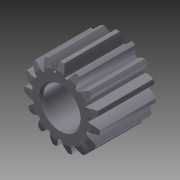
# Autodesk Inventor part: 15T Gear P60 Pinion Gear
Saved by Autodesk Inventor 2014 SP1 (Build 180222100, 222)
## iProperties
Created: 2013-05-05
Part Number: 15T Gear P60 Pinion Gear
Material: Steel
Document SubType Name: Modeling
Designer: Moses
Categories: <?xml version="1.0" encoding="UTF-16"?> <MemberInstance><Categories><FamilyTemplate><FamilyTemplateParameter ValueType="xs:double" Id="1" ObjectReferenceKey="da_z" ObjectType="kUserParameterObject"/><FamilyTemplateParameter ValueType="xs:double" Id="2" ObjectReferenceKey="da_b" ObjectType="kUserParameterObject"/><FamilyTemplateParameter ValueType="xs:double" Id="3" ObjectReferenceKey="da_beta" ObjectType="kUserParameterObject"/><FamilyTemplateParameter ValueType="xs:double" Id="4" ObjectReferenceKey="da_da" ObjectType="kUserParameterObject"/><FamilyTemplateParameter ValueType="xs:double" Id="5" ObjectReferenceKey="da_aw" ObjectType="kUserParameterObject"/><FamilyTemplateParameter ValueType="xs:string" Id="6" ObjectReferenceKey="EAIAABAAAAC/AAAAAAAAAIAAAAAAAAAA" ObjectType="83910656" SubObjectId="SurfaceGeometry"/></FamilyTemplate><ParamToTemplateMap><ParamToTemplate CategoryParameter="//CategoryParameter[@InternalName='046C89C9-8512-4d59-83FE-43B91F4F132A']" TemplateParameter="1"/><ParamToTemplate CategoryParameter="//CategoryParameter[@InternalName='2552DF32-E462-4b46-AEBF-C6C7768E72AC']" TemplateParameter="2"/><ParamToTemplate CategoryParameter="//CategoryParameter[@InternalName='C9EE641D-15FC-4fae-A226-E94C4372FDD7']" TemplateParameter="3"/><ParamToTemplate><ParamToTemplate CategoryParameter="//CategoryParameter[@InternalName='00B6519A-459B-49c7-AD84-2E56D39A5744']" ConstantValue="0.000000"/></ParamToTemplate><ParamToTemplate><ParamToTemplate CategoryParameter="//CategoryParameter[@InternalName='04B31F0E-C7A6-4894-AA32-9629BEFACF47']" ConstantValue="1.000000"/></ParamToTemplate><ParamToTemplate><ParamToTemplate CategoryParameter="//CategoryParameter[@InternalName='43CBEC2E-7847-49e7-A936-2F7889FCB2D9']" ConstantValue="0.250000"/></ParamToTemplate><ParamToTemplate><ParamToTemplate CategoryParameter="//CategoryParameter[@InternalName='B1EFC894-105D-4ebd-86BF-FA20ED196853']" ConstantValue="0.350000"/></ParamToTemplate><ParamToTemplate><ParamToTemplate CategoryParameter="//CategoryParameter[@InternalName='51175063-3D10-4879-93E8-6246FE8B403D']" ConstantValue="2060110000.000000"/></ParamToTemplate><ParamToTemplate><ParamToTemplate CategoryParameter="//CategoryParameter[@InternalName='A3A52E27-4454-46a9-B0BD-C932399B70AF']" ConstantValue="0.300000"/></ParamToTemplate><ParamToTemplate><ParamToTemplate CategoryParameter="//CategoryParameter[@InternalName='91B76062-C214-41d9-B1B9-14D2AB99603D']" ConstantValue="0.060000"/></ParamToTemplate><ParamToTemplate><ParamToTemplate CategoryParameter="//CategoryParameter[@InternalName='374E806E-8B8A-4dda-A9AA-1039D6500AD2']" ConstantValue="16.666667"/></ParamToTemplate><ParamToTemplate><ParamToTemplate CategoryParameter="//CategoryParameter[@InternalName='2D373A89-B862-43d6-8D0B-0CBF12AB9F6C']" ConstantValue="0.349066"/></ParamToTemplate><ParamToTemplate CategoryParameter="//CategoryParameter[@InternalName='37777632-D6A2-4fac-9D53-DB8ACD95C989']" TemplateParameter="4"/><ParamToTemplate CategoryParameter="//CategoryParameter[@InternalName='FD1017F1-B727-4f7e-9707-0F86F1FF9423']" TemplateParameter="5"/><ParamToTemplate><ParamToTemplate CategoryParameter="//CategoryParameter[@InternalName='9E1B4470-B2D3-4ff1-B813-535BB4CDF51A']" ConstantValue="3520790.000000"/></ParamToTemplate><ParamToTemplate><ParamToTemplate CategoryParameter="//CategoryParameter[@InternalName='F8452263-BFF6-458c-9FB1-07C4B99E95CD']" ConstantValue="11389170.000000"/></ParamToTemplate><ParamToTemplate><ParamToTemplate CategoryParameter="//CategoryParameter[@InternalName='3E3BB259-FD49-497f-8171-6EBC954A3479']" ConstantValue="2.000000"/></ParamToTemplate><ParamToTemplate CategoryParameter="//CategoryParameter[@InternalName='27C3BAF2-7550-4e4b-AE2C-0DB134B7D9B7']" TemplateParameter="6"/></ParamToTemplateMap><Category DisplayName="Gear" InternalName="DC85795E-93AB-48d5-8EEE-5A27447B64BD" Mnemonic="Gear"><CategoryParameter DisplayName="z" InternalName="046C89C9-8512-4d59-83FE-43B91F4F132A" Mnemonic="z"/><CategoryParameter DisplayName="b" InternalName="2552DF32-E462-4b46-AEBF-C6C7768E72AC" Mnemonic="b"/><CategoryParameter DisplayName="||b|" InternalName="C9EE641D-15FC-4fae-A226-E94C4372FDD7" Mnemonic="beta"/><CategoryParameter DisplayName="x" InternalName="00B6519A-459B-49c7-AD84-2E56D39A5744" Mnemonic="x"/><CategoryParameter DisplayName="a*" InternalName="04B31F0E-C7A6-4894-AA32-9629BEFACF47" Mnemonic="a"/><CategoryParameter DisplayName="c*" InternalName="43CBEC2E-7847-49e7-A936-2F7889FCB2D9" Mnemonic="c"/><CategoryParameter DisplayName="r|.f|*" InternalName="B1EFC894-105D-4ebd-86BF-FA20ED196853" Mnemonic="rf"/><CategoryParameter DisplayName="E" InternalName="51175063-3D10-4879-93E8-6246FE8B403D" Mnemonic="E"/><CategoryParameter DisplayName="||m|" InternalName="A3A52E27-4454-46a9-B0BD-C932399B70AF" Mnemonic="mi"/><Category DisplayName="SpurGear" InternalName="26C5A22E-A91E-4dfd-A3B3-23CCAFAE1764" Mnemonic="SpurGear"><CategoryParameter DisplayName="m" InternalName="91B76062-C214-41d9-B1B9-14D2AB99603D" Mnemonic="m"/><CategoryParameter DisplayName="P" InternalName="374E806E-8B8A-4dda-A9AA-1039D6500AD2" Mnemonic="PP"/><CategoryParameter DisplayName="||a|" InternalName="2D373A89-B862-43d6-8D0B-0CBF12AB9F6C" Mnemonic="alpha"/><CategoryParameter DisplayName="d|.a|" InternalName="37777632-D6A2-4fac-9D53-DB8ACD95C989" Mnemonic="da"/><CategoryParameter DisplayName="a|.w|" InternalName="FD1017F1-B727-4f7e-9707-0F86F1FF9423" Mnemonic="aw"/><CategoryParameter DisplayName="||s||.Flim|" InternalName="9E1B4470-B2D3-4ff1-B813-535BB4CDF51A" Mnemonic="sFlim"/><CategoryParameter DisplayName="||s||.Hlim|" InternalName="F8452263-BFF6-458c-9FB1-07C4B99E95CD" Mnemonic="sHlim"/><CategoryParameter DisplayName="type" InternalName="3E3BB259-FD49-497f-8171-6EBC954A3479" Mnemonic="type"/><CategoryParameter DisplayName="PitchDiameter" InternalName="27C3BAF2-7550-4e4b-AE2C-0DB134B7D9B7" Mnemonic="IDS_PITCHDIAM"/></Category></Category></Categories></MemberInstance>
Density: 7.85 g/cm^3
Mass: 2.25857 g
Surface Area: 4.2591 cm^2
Volume: 0.287716 cm^3
Appearance: Steel
CustomPartVersion: 1
Author: Moses
Autodesk Inventor part; units mm, degrees
sketch "Sketch1" plane through (0, 0, 0) normal (0, 0, 1) x (1, 0, 0)
  circle A0 centre (0, 0) radius 5.1
  dimension "d0" = 10.2
  constraints: 1 centre point
  measures "d0" diameter of A0
extrude "Extrusion1" add sketch "Sketch1" along normal mid plane 5
sketch "Sketch2" plane through (0, 0, -2.5) normal (0, 0, -1) x (-1, 0, 0)
  circle A0 centre (0, 0) radius 5.1 projected
  circle A1 centre (0, 0) radius 4.5
  dimension "d3" = 9
  constraints: 1 centre point, 1 coincident
  measures "d3" diameter of A1
surface extrude "Pitch Diameter" sketch "Sketch2" against normal through all shown no curves A1
ref_plane "Work Plane1" through (0, 0, 0) normal (1, 0, 0) x (0, 1, 0)
ref_plane "Work Plane2" through (0, 0, 0) normal (0.9781476, 0.2079117, 0) x (0, 0, 1)
ref_plane "Work Plane3" through (0, 0, 0) normal (0, 0, -1) x (-1, 0, 0)
spur gear teeth "Spur Gear" teeth 15 pitch diameter 9 tip diameter 10.2 root diameter 7.5 face width 5 start plane through (0, 0, -2.5) normal (0, 0, -1) x (-1, 0, 0)
sketch "Sketch3" plane through (0, 0, 2.5) normal (0, 0, 1) x (1, 0, 0)
  arc A0 (-1.8277, 4.7613) -> (-2.3154, 4.5441) centre (0, 0) ccw projected
  circle A1 centre (0, 0) radius 2.5
  dimension "d20" = 5
  constraints: 1 centre point, 1 coincident
  measures "d20" diameter of A1
extrude "Extrusion2" cut sketch "Sketch3" against normal through all
chamfer "Chamfer3" distance 1 angle 15 15 edges at (4.8504, 1.576, -2.5) (5.0721, -0.5331, -2.5) (3.79, 3.4126, -2.5) (4.4167, -2.55, -2.5) (2.0744, 4.6591, -2.5) (2.9977, -4.126, -2.5) (0, 5.1, -2.5) (1.0603, -4.9886, -2.5) (-2.0744, 4.6591, -2.5) (-1.0603, -4.9886, -2.5) (-3.79, 3.4126, -2.5) (-2.9977, -4.126, -2.5) (-4.8504, 1.576, -2.5) (-4.4167, -2.55, -2.5) (-5.0721, -0.5331, -2.5) measured on face at (-0.1004, 3.2965, -2.5)
sketch "Sketch4" plane through (0, 0, 2.5) normal (0, 0, 1) x (1, 0, 0)
  arc A0 (-2.36, 2.9143) -> (-3.6062, 3.6062) centre (-5.0149, -0.3993) ccw projected
  arc A1 (-3.6062, 3.6062) -> (-3.9634, 3.2095) centre (0, 0) ccw projected
  arc A2 (-3.9634, 3.2095) -> (-3.145, 2.0424) centre (-0.1271, 5.0291) ccw projected
  arc A3 (-3.145, 2.0424) -> (-3.3413, 1.7025) centre (0, 0) ccw projected
  arc A4 (-3.3413, 1.7025) -> (-4.7613, 1.8277) centre (-4.4189, -2.4045) ccw projected
  arc A5 (-4.7613, 1.8277) -> (-4.9262, 1.32) centre (0, 0) ccw projected
  arc A6 (-4.9262, 1.32) -> (-3.7038, 0.5866) centre (-2.1617, 4.5426) ccw projected
  arc A7 (-3.7038, 0.5866) -> (-3.7449, 0.1963) centre (0, 0) ccw projected
  arc A8 (-3.7449, 0.1963) -> (-5.093, -0.2669) centre (-3.0589, -3.9939) ccw projected
  arc A9 (-5.093, -0.2669) -> (-5.0372, -0.7978) centre (0, 0) ccw projected
  arc A10 (-5.0372, -0.7978) -> (-3.6222, -0.9706) centre (-3.8224, 3.2707) ccw projected
  arc A11 (-3.6222, -0.9706) -> (-3.5009, -1.3439) centre (0, 0) ccw projected
  arc A12 (-3.5009, -1.3439) -> (-4.5441, -2.3154) centre (-1.17, -4.8928) ccw projected
  arc A13 (-4.5441, -2.3154) -> (-4.2772, -2.7777) centre (0, 0) ccw projected
  arc A14 (-4.2772, -2.7777) -> (-2.9143, -2.36) centre (-4.8223, 1.4332) ccw projected
  arc A15 (-2.9143, -2.36) -> (-2.6517, -2.6517) centre (0, 0) ccw projected
  arc A16 (-2.6517, -2.6517) -> (-3.2095, -3.9634) centre (0.9213, -4.9457) ccw projected
  arc A17 (-3.2095, -3.9634) -> (-2.7777, -4.2772) centre (0, 0) ccw projected
  arc A18 (-2.7777, -4.2772) -> (-1.7025, -3.3413) centre (-4.9883, -0.6521) ccw projected
  arc A19 (-1.7025, -3.3413) -> (-1.3439, -3.5009) centre (0, 0) ccw projected
  arc A20 (-1.3439, -3.5009) -> (-1.32, -4.9262) centre (2.8532, -4.1434) ccw projected
  arc A21 (-1.32, -4.9262) -> (-0.7978, -5.0372) centre (0, 0) ccw projected
  arc A22 (-0.7978, -5.0372) -> (-0.1963, -3.7449) centre (-4.2918, -2.6247) ccw projected
  arc A23 (-0.1963, -3.7449) -> (0.1963, -3.7449) centre (0, 0) ccw projected
  arc A24 (0.1963, -3.7449) -> (0.7978, -5.0372) centre (4.2918, -2.6247) ccw projected
  arc A25 (0.7978, -5.0372) -> (1.32, -4.9262) centre (0, 0) ccw projected
  arc A26 (1.32, -4.9262) -> (1.3439, -3.5009) centre (-2.8532, -4.1434) ccw projected
  arc A27 (1.3439, -3.5009) -> (1.7025, -3.3413) centre (0, 0) ccw projected
  arc A28 (1.7025, -3.3413) -> (2.7777, -4.2772) centre (4.9883, -0.6521) ccw projected
  arc A29 (2.7777, -4.2772) -> (3.2095, -3.9634) centre (0, 0) ccw projected
  arc A30 (3.2095, -3.9634) -> (2.6517, -2.6517) centre (-0.9213, -4.9457) ccw projected
  arc A31 (2.6517, -2.6517) -> (2.9143, -2.36) centre (0, 0) ccw projected
  arc A32 (2.9143, -2.36) -> (4.2772, -2.7777) centre (4.8223, 1.4332) ccw projected
  arc A33 (4.2772, -2.7777) -> (4.5441, -2.3154) centre (0, 0) ccw projected
  arc A34 (4.5441, -2.3154) -> (3.5009, -1.3439) centre (1.17, -4.8928) ccw projected
  arc A35 (3.5009, -1.3439) -> (3.6222, -0.9706) centre (0, 0) ccw projected
  arc A36 (3.6222, -0.9706) -> (5.0372, -0.7978) centre (3.8224, 3.2707) ccw projected
  arc A37 (5.0372, -0.7978) -> (5.093, -0.2669) centre (0, 0) ccw projected
  arc A38 (5.093, -0.2669) -> (3.7449, 0.1963) centre (3.0589, -3.9939) ccw projected
  arc A39 (3.7449, 0.1963) -> (3.7038, 0.5866) centre (0, 0) ccw projected
  arc A40 (3.7038, 0.5866) -> (4.9262, 1.32) centre (2.1617, 4.5426) ccw projected
  arc A41 (4.9262, 1.32) -> (4.7613, 1.8277) centre (0, 0) ccw projected
  arc A42 (4.7613, 1.8277) -> (3.3413, 1.7025) centre (4.4189, -2.4045) ccw projected
  arc A43 (3.3413, 1.7025) -> (3.145, 2.0424) centre (0, 0) ccw projected
  arc A44 (3.145, 2.0424) -> (3.9634, 3.2095) centre (0.1271, 5.0291) ccw projected
  arc A45 (3.9634, 3.2095) -> (3.6062, 3.6062) centre (0, 0) ccw projected
  arc A46 (3.6062, 3.6062) -> (2.36, 2.9143) centre (5.0149, -0.3993) ccw projected
  arc A47 (2.36, 2.9143) -> (2.0424, 3.145) centre (0, 0) ccw projected
  arc A48 (2.0424, 3.145) -> (2.3154, 4.5441) centre (-1.9294, 4.6461) ccw projected
  arc A49 (2.3154, 4.5441) -> (1.8277, 4.7613) centre (0, 0) ccw projected
  arc A50 (1.8277, 4.7613) -> (0.9706, 3.6222) centre (4.7437, 1.675) ccw projected
  arc A51 (0.9706, 3.6222) -> (0.5866, 3.7038) centre (0, 0) ccw projected
  arc A52 (0.5866, 3.7038) -> (0.2669, 5.093) centre (-3.6523, 3.4596) ccw projected
  arc A53 (0.2669, 5.093) -> (-0.2669, 5.093) centre (0, 0) ccw projected
  arc A54 (-0.2669, 5.093) -> (-0.5866, 3.7038) centre (3.6523, 3.4596) ccw projected
  arc A55 (-0.5866, 3.7038) -> (-0.9706, 3.6222) centre (0, 0) ccw projected
  arc A56 (-0.9706, 3.6222) -> (-1.8277, 4.7613) centre (-4.7437, 1.675) ccw projected
  arc A57 (-1.8277, 4.7613) -> (-2.3154, 4.5441) centre (0, 0) ccw projected
  arc A58 (-2.3154, 4.5441) -> (-2.0424, 3.145) centre (1.9294, 4.6461) ccw projected
  arc A59 (-2.0424, 3.145) -> (-2.36, 2.9143) centre (0, 0) ccw projected
  circle A60 centre (0, 0) radius 2.5 projected
  arc A61 (-2.36, 2.9143) -> (-3.6062, 3.6062) centre (-5.0149, -0.3993) ccw projected
  arc A62 (-3.6062, 3.6062) -> (-3.9634, 3.2095) centre (0, 0) ccw projected
  arc A63 (-3.9634, 3.2095) -> (-3.145, 2.0424) centre (-0.1271, 5.0291) ccw projected
  arc A64 (-3.145, 2.0424) -> (-3.3413, 1.7025) centre (0, 0) ccw projected
  arc A65 (-3.3413, 1.7025) -> (-4.7613, 1.8277) centre (-4.4189, -2.4045) ccw projected
  arc A66 (-4.7613, 1.8277) -> (-4.9262, 1.32) centre (0, 0) ccw projected
  arc A67 (-4.9262, 1.32) -> (-3.7038, 0.5866) centre (-2.1617, 4.5426) ccw projected
  arc A68 (-3.7038, 0.5866) -> (-3.7449, 0.1963) centre (0, 0) ccw projected
  arc A69 (-3.7449, 0.1963) -> (-5.093, -0.2669) centre (-3.0589, -3.9939) ccw projected
  arc A70 (-5.093, -0.2669) -> (-5.0372, -0.7978) centre (0, 0) ccw projected
  arc A71 (-5.0372, -0.7978) -> (-3.6222, -0.9706) centre (-3.8224, 3.2707) ccw projected
  arc A72 (-3.6222, -0.9706) -> (-3.5009, -1.3439) centre (0, 0) ccw projected
  arc A73 (-3.5009, -1.3439) -> (-4.5441, -2.3154) centre (-1.17, -4.8928) ccw projected
  arc A74 (-4.5441, -2.3154) -> (-4.2772, -2.7777) centre (0, 0) ccw projected
  arc A75 (-4.2772, -2.7777) -> (-2.9143, -2.36) centre (-4.8223, 1.4332) ccw projected
  arc A76 (-2.9143, -2.36) -> (-2.6517, -2.6517) centre (0, 0) ccw projected
  arc A77 (-2.6517, -2.6517) -> (-3.2095, -3.9634) centre (0.9213, -4.9457) ccw projected
  arc A78 (-3.2095, -3.9634) -> (-2.7777, -4.2772) centre (0, 0) ccw projected
  arc A79 (-2.7777, -4.2772) -> (-1.7025, -3.3413) centre (-4.9883, -0.6521) ccw projected
  arc A80 (-1.7025, -3.3413) -> (-1.3439, -3.5009) centre (0, 0) ccw projected
  arc A81 (-1.3439, -3.5009) -> (-1.32, -4.9262) centre (2.8532, -4.1434) ccw projected
  arc A82 (-1.32, -4.9262) -> (-0.7978, -5.0372) centre (0, 0) ccw projected
  arc A83 (-0.7978, -5.0372) -> (-0.1963, -3.7449) centre (-4.2918, -2.6247) ccw projected
  arc A84 (-0.1963, -3.7449) -> (0.1963, -3.7449) centre (0, 0) ccw projected
  arc A85 (0.1963, -3.7449) -> (0.7978, -5.0372) centre (4.2918, -2.6247) ccw projected
  arc A86 (0.7978, -5.0372) -> (1.32, -4.9262) centre (0, 0) ccw projected
  arc A87 (1.32, -4.9262) -> (1.3439, -3.5009) centre (-2.8532, -4.1434) ccw projected
  arc A88 (1.3439, -3.5009) -> (1.7025, -3.3413) centre (0, 0) ccw projected
  arc A89 (1.7025, -3.3413) -> (2.7777, -4.2772) centre (4.9883, -0.6521) ccw projected
  arc A90 (2.7777, -4.2772) -> (3.2095, -3.9634) centre (0, 0) ccw projected
  arc A91 (3.2095, -3.9634) -> (2.6517, -2.6517) centre (-0.9213, -4.9457) ccw projected
  arc A92 (2.6517, -2.6517) -> (2.9143, -2.36) centre (0, 0) ccw projected
  arc A93 (2.9143, -2.36) -> (4.2772, -2.7777) centre (4.8223, 1.4332) ccw projected
  arc A94 (4.2772, -2.7777) -> (4.5441, -2.3154) centre (0, 0) ccw projected
  arc A95 (4.5441, -2.3154) -> (3.5009, -1.3439) centre (1.17, -4.8928) ccw projected
  arc A96 (3.5009, -1.3439) -> (3.6222, -0.9706) centre (0, 0) ccw projected
  arc A97 (3.6222, -0.9706) -> (5.0372, -0.7978) centre (3.8224, 3.2707) ccw projected
  arc A98 (5.0372, -0.7978) -> (5.093, -0.2669) centre (0, 0) ccw projected
  arc A99 (5.093, -0.2669) -> (3.7449, 0.1963) centre (3.0589, -3.9939) ccw projected
  arc A100 (3.7449, 0.1963) -> (3.7038, 0.5866) centre (0, 0) ccw projected
  arc A101 (3.7038, 0.5866) -> (4.9262, 1.32) centre (2.1617, 4.5426) ccw projected
  arc A102 (4.9262, 1.32) -> (4.7613, 1.8277) centre (0, 0) ccw projected
  arc A103 (4.7613, 1.8277) -> (3.3413, 1.7025) centre (4.4189, -2.4045) ccw projected
  arc A104 (3.3413, 1.7025) -> (3.145, 2.0424) centre (0, 0) ccw projected
  arc A105 (3.145, 2.0424) -> (3.9634, 3.2095) centre (0.1271, 5.0291) ccw projected
  arc A106 (3.9634, 3.2095) -> (3.6062, 3.6062) centre (0, 0) ccw projected
  arc A107 (3.6062, 3.6062) -> (2.36, 2.9143) centre (5.0149, -0.3993) ccw projected
  arc A108 (2.36, 2.9143) -> (2.0424, 3.145) centre (0, 0) ccw projected
  arc A109 (2.0424, 3.145) -> (2.3154, 4.5441) centre (-1.9294, 4.6461) ccw projected
  arc A110 (2.3154, 4.5441) -> (1.8277, 4.7613) centre (0, 0) ccw projected
  arc A111 (1.8277, 4.7613) -> (0.9706, 3.6222) centre (4.7437, 1.675) ccw projected
  arc A112 (0.9706, 3.6222) -> (0.5866, 3.7038) centre (0, 0) ccw projected
  arc A113 (0.5866, 3.7038) -> (0.2669, 5.093) centre (-3.6523, 3.4596) ccw projected
  arc A114 (0.2669, 5.093) -> (-0.2669, 5.093) centre (0, 0) ccw projected
  arc A115 (-0.2669, 5.093) -> (-0.5866, 3.7038) centre (3.6523, 3.4596) ccw projected
  arc A116 (-0.5866, 3.7038) -> (-0.9706, 3.6222) centre (0, 0) ccw projected
  arc A117 (-0.9706, 3.6222) -> (-1.8277, 4.7613) centre (-4.7437, 1.675) ccw projected
  arc A118 (-1.8277, 4.7613) -> (-2.3154, 4.5441) centre (0, 0) ccw projected
  arc A119 (-2.3154, 4.5441) -> (-2.0424, 3.145) centre (1.9294, 4.6461) ccw projected
  arc A120 (-2.0424, 3.145) -> (-2.36, 2.9143) centre (0, 0) ccw projected
extrude "Extrusion3" add sketch "Sketch4" along normal blind 3
chamfer "Chamfer2" distance 1 angle 15 15 edges at (-2.0744, 4.6591, 5.5) (0, 5.1, 5.5) (-3.79, 3.4126, 5.5) (-4.8504, 1.576, 5.5) (-5.0721, -0.5331, 5.5) (-4.4167, -2.55, 5.5) (-2.9977, -4.126, 5.5) (-1.0603, -4.9886, 5.5) (1.0603, -4.9886, 5.5) (2.9977, -4.126, 5.5) (4.4167, -2.55, 5.5) (5.0721, -0.5331, 5.5) (4.8504, 1.576, 5.5) (3.79, 3.4126, 5.5) (2.0744, 4.6591, 5.5) measured on face at (-0.1004, 3.2965, 5.5)
chamfer "Chamfer1" distance 0.254 angle 45 2 edges at (-2.5, 0, -2.5) (-2.5, 0, 5.5)
equation "\"d0\" = da_da"
equation "\"d1\" = da_b"
equation "\"d3\" = da_dw"
equation "\"d15\" = da_aw"
equation "\"d19\" = da_aw"
equation "\"da_da\" = 10.2"
equation "\"da_b\" = 5"
equation "\"da_dw\" = 9"
equation "\"da_aw\" = 9"
body "Solid1"
body "Srf1"
